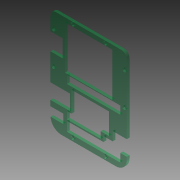
# Autodesk Inventor part: beagle_spacer_top
Saved by Autodesk Inventor 2014 (Build 180170000, 170)
## iProperties
Created: 2013-06-20
Part Number: beagle_spacer_top
Document SubType Name: Modeling
Designer: Administrator
Density: 1 g/cm^3
Mass: 13.5107 g
Surface Area: 121.813 cm^2
Volume: 13.5107 cm^3
Material: Generic
Appearance: Clear - Green 1
Author: Administrator
Autodesk Inventor part; units mm, degrees
ref_plane "YZ Plane" through (0, 0, 0) normal (1, 0, 0) x (0, 1, 0)
ref_plane "XZ Plane" through (0, 0, 0) normal (0, 1, 0) x (-1, 0, 0)
ref_plane "XY Plane" through (0, 0, 0) normal (0, 0, 1) x (1, 0, 0)
sketch "Sketch1" plane through (0, 0, 0) normal (0, 0, 1) x (1, 0, 0)
  line L0 (9.8795, 48.1994) -> (9.8795, -53.4006)
  line L1 (16.2295, 54.5494) -> (92.4295, 54.5494)
  line L2 (98.7795, 48.1994) -> (98.7795, -53.4006)
  line L3 (22.5795, -66.1006) -> (86.0795, -66.1006)
  arc A0 (9.8795, -53.4006) -> (22.5795, -66.1006) centre (22.5795, -53.4006) ccw
  arc A1 (16.2295, 54.5494) -> (9.8795, 48.1994) centre (16.2295, 48.1994) ccw
  arc A2 (98.7795, 48.1994) -> (92.4295, 54.5494) centre (92.4295, 48.1994) ccw
  arc A3 (86.0795, -66.1006) -> (98.7795, -53.4006) centre (86.0795, -53.4006) ccw
  point P0 (0, 0)
  dimension "d0" = 12.7
  dimension "d1" = 6.35
  dimension "d2" = 120.65
  dimension "d3" = 88.9
  constraints: 8 end point, 8 point on circle, 8 tangent, 4 centre point, 2 equal radius, 1 horizontal, 1 vertical
  measures "d0" radius of A0
  measures "d1" radius of A1
  measures "d2" distance between parallel lines of L3 L1
  measures "d3" distance between parallel lines of L2 L0
extrude "Extrusion1" add sketch "Sketch1" along normal blind 3.175
sketch "Sketch2" plane through (0, 0, 3.175) normal (0, 0, 1) x (1, 0, 0)
  line L0 (9.8795, -53.4006) -> (9.8795, 48.1994) projected
  line L1 (98.7795, 48.1994) -> (98.7795, -53.4006) projected
  line L2 (16.2295, 54.5494) -> (92.4295, 54.5494) projected
  line L3 (26.6435, 49.4694) -> (82.0155, 49.4694)
  line L4 (82.0155, 49.4694) -> (82.0155, -1.3306)
  line L5 (82.0155, -1.3306) -> (26.6435, -1.3306)
  line L6 (26.6435, -1.3306) -> (26.6435, 49.4694)
  point P0 (0, 0)
  dimension "d13" = 16.764
  dimension "d14" = 16.764
  dimension "d15" = 5.08
  dimension "d16" = 55.88
  constraints: 8 end point
  measures "d13" distance between parallel lines of L0 L6
  measures "d14" distance between parallel lines of L1 L4
  measures "d15" distance between parallel lines of L2 L3
  measures "d16" distance between parallel lines of L5 L2
extrude "Extrusion2" cut sketch "Sketch2" against normal through all
sketch "Sketch3" plane through (0, 0, 3.175) normal (0, 0, 1) x (1, 0, 0)
  line L0 (9.8795, -53.4006) -> (9.8795, 48.1994) projected
  line L1 (86.0795, -66.1006) -> (22.5795, -66.1006) projected
  line L2 (9.8795, -19.4408) -> (32.7395, -19.4408)
  line L3 (32.7395, -19.4408) -> (32.7395, -37.2208)
  line L4 (32.7395, -37.2208) -> (9.8795, -37.2208)
  point P0 (0, 0)
  dimension "d20" = 28.8798
  dimension "d21" = 46.6598
  dimension "d22" = 22.86
  constraints: 6 end point, 2 point on line
  measures "d20" distance between parallel lines of L4 L1
  measures "d21" distance between parallel lines of L1 L2
  measures "d22" distance between parallel lines of L3 L0
extrude "Extrusion3" cut sketch "Sketch3" against normal through all
sketch "Sketch4" plane through (0, 0, 3.175) normal (0, 0, 1) x (1, 0, 0)
  line L0 (9.8795, -53.4006) -> (9.8795, -37.2208) projected
  arc A0 (9.8795, -53.4006) -> (22.5795, -66.1006) centre (22.5795, -53.4006) ccw projected
  line L1 (86.0795, -66.1006) -> (22.5795, -66.1006) projected
  line L2 (24.8655, -43.5708) -> (24.8655, -54.1626)
  line L3 (24.8655, -43.5708) -> (9.8795, -43.5708)
  line L4 (24.8655, -54.1626) -> (9.9024, -54.1626)
  point P0 (0, 0)
  dimension "d26" = 22.5298
  dimension "d27" = 14.986
  dimension "d28" = 11.938
  constraints: 6 end point, 1 horizontal, 1 point on circle, 1 point on line, 1 vertical
  measures "d26" distance between parallel lines of L1 L3
  measures "d27" distance between parallel lines of L0 L2
  measures "d28" distance between parallel lines of L1 L4
extrude "Extrusion4" cut sketch "Sketch4" against normal through all
sketch "Sketch5" plane through (0, 0, 3.175) normal (0, 0, 1) x (1, 0, 0)
  line L0 (86.0795, -66.1006) -> (22.5795, -66.1006) projected
  line L1 (9.8795, -19.4408) -> (9.8795, 48.1994) projected
  line L2 (9.8795, -43.5708) -> (9.8795, -37.2208) projected
  line L3 (28.9295, -2.1688) -> (91.1595, -2.1688)
  line L4 (91.1595, -2.1688) -> (91.1595, -11.5668)
  line L5 (91.1595, -11.5668) -> (28.9295, -11.5668)
  line L6 (28.9295, -11.5668) -> (28.9295, -2.1688)
  line L7 (28.9295, -50.4288) -> (91.1595, -50.4288)
  line L8 (91.1595, -50.4288) -> (91.1595, -59.8268)
  line L9 (91.1595, -59.8268) -> (28.9295, -59.8268)
  line L10 (28.9295, -59.8268) -> (28.9295, -50.4288)
  point P0 (0, 0)
  dimension "d31" = 54.5338
  dimension "d32" = 9.398
  dimension "d33" = 62.23
  dimension "d34" = 19.05
  dimension "d35" = 19.05
  dimension "d36" = 6.2738
  constraints: 16 end point, 2 equal length
  measures "d31" distance between parallel lines of L0 L5
  measures "d32" distance between parallel lines of L3 L5
  measures "d33" distance of L4.end L5.end
  measures "d34" distance between parallel lines of L1 L6
  measures "d35" distance between parallel lines of L2 L10
  measures "d36" distance between parallel lines of L9 L0
extrude "Extrusion5" cut sketch "Sketch5" against normal through all
sketch "Sketch6" plane through (0, 0, 3.175) normal (0, 0, 1) x (1, 0, 0)
  line L0 (71.6015, -11.5668) -> (28.9295, -11.5668)
  line L1 (28.9295, -50.4288) -> (71.6015, -50.4288)
  line L2 (71.6015, -50.4288) -> (71.6015, -11.5668)
  line L3 (28.9295, -59.8268) -> (28.9295, -50.4288) projected
  line L4 (28.9295, -11.5668) -> (28.9295, -50.4288)
  line L5 (28.9295, -47.2538) -> (68.4265, -47.2538)
  line L6 (9.8795, -19.4408) -> (32.7395, -19.4408) projected
  line L7 (32.7395, -19.4408) -> (32.7395, -37.2208) projected
  line L8 (32.7395, -37.2208) -> (9.8795, -37.2208) projected
  line L9 (28.9295, -17.8533) -> (34.327, -17.8533)
  line L10 (34.327, -17.8533) -> (34.327, -38.8083)
  line L11 (34.327, -38.8083) -> (28.9295, -38.8083)
  line L12 (91.1595, -11.5668) -> (28.9295, -11.5668) projected
  line L13 (28.9295, -50.4288) -> (91.1595, -50.4288) projected
  line L14 (91.1595, -50.4288) -> (91.1595, -42.8088)
  line L15 (91.1595, -42.8088) -> (71.6015, -42.8088)
  line L16 (28.9295, -14.7418) -> (71.6015, -14.7418)
  line L17 (28.9295, -48.8413) -> (71.6015, -48.8413)
  line L18 (68.4265, -47.2538) -> (68.4265, -39.6338)
  line L19 (68.4265, -39.6338) -> (71.6015, -39.6338)
  line L20 (91.1595, -50.4288) -> (71.6015, -50.4288)
  line L21 (98.7795, 48.1994) -> (98.7795, -53.4006) projected
  line L22 (34.327, -17.8533) -> (34.327, -14.7418)
  point P0 (0, 0)
  dimension "d46" = 3.175
  dimension "d49" = 1.5875
  dimension "d50" = 1.5875
  dimension "d51" = 1.5875
  dimension "d54" = 7.62
  dimension "d55" = 3.175
  dimension "d57" = 1.5875
  dimension "d58" = 3.175
  dimension "d61" = 3.175
  dimension "d72" = 27.178
  constraints: 32 end point, 11 point on line, 5 vertical, 2 collinear
  measures "d46" distance between parallel lines of L1 L5
  measures "d49" distance between parallel lines of L8 L11
  measures "d50" distance between parallel lines of L10 L7
  measures "d51" distance between parallel lines of L6 L9
  measures "d54" distance between parallel lines of L13 L15
  measures "d55" distance between parallel lines of L12 L16
  measures "d57" distance between parallel lines of L1 L17
  measures "d58" distance between parallel lines of L15 L19
  measures "d61" distance between parallel lines of L2 L18
  measures "d72" distance between parallel lines of L21 L2
extrude "Extrusion11" cut sketch "Sketch6" against normal through all contours L2 L19 L18 L5 L4 L11 L10 L22 L16 | L15 L14 L13 L2 | L2 L1 L4 L17
sketch "Sketch7" plane through (0, 0, 3.175) normal (0, 0, 1) x (1, 0, 0)
  line L0 (71.6015, -14.7418) -> (71.6015, -39.6338) projected
  line L1 (71.6015, -14.7418) -> (77.9515, -14.7418)
  line L2 (77.9515, -14.7418) -> (77.9515, -39.6338)
  line L3 (77.9515, -39.6338) -> (71.6015, -39.6338)
  point P0 (0, 0)
  dimension "d64" = 6.35
  constraints: 6 end point, 2 horizontal
  measures "d64" distance between parallel lines of L2 L0
extrude "Extrusion12" cut sketch "Sketch7" against normal through all
sketch "Sketch8" plane through (0, 0, 3.175) normal (0, 0, 1) x (1, 0, 0)
  line L0 (86.0795, -66.1006) -> (22.5795, -66.1006) projected
  line L1 (98.7795, 48.1994) -> (98.7795, -53.4006) projected
  line L2 (82.2695, -32.3948) -> (98.7795, -32.3948)
  line L3 (98.7795, -32.3948) -> (98.7795, -50.1748)
  line L4 (98.7795, -50.1748) -> (82.2695, -50.1748)
  line L5 (82.2695, -50.1748) -> (82.2695, -32.3948)
  point P0 (0, 0)
  dimension "d67" = 15.9258
  dimension "d68" = 17.78
  dimension "d69" = 16.51
  constraints: 8 end point, 1 collinear, 1 horizontal, 1 vertical
  measures "d67" distance between parallel lines of L0 L4
  measures "d68" distance of L4.end L2.start
  measures "d69" distance of L2.start L2.end
extrude "Extrusion13" cut sketch "Sketch8" against normal through all
sketch "Sketch9" plane through (0, 0, 3.175) normal (0, 0, 1) x (1, 0, 0)
  line L0 (98.7795, 48.1994) -> (98.7795, -32.3948) projected
  line L1 (16.2295, 54.5494) -> (92.4295, 54.5494) projected
  line L2 (9.8795, -19.4408) -> (9.8795, 48.1994) projected
  line L3 (86.0795, -66.1006) -> (22.5795, -66.1006) projected
  line L4 (36.2694, 49.7107) -> (34.2897, 49.7107)
  line L5 (34.2897, 49.7107) -> (33.2998, 51.4252)
  line L6 (33.2998, 51.4252) -> (34.2897, 53.1397)
  line L7 (34.2897, 53.1397) -> (36.2694, 53.1397)
  line L8 (36.2694, 53.1397) -> (37.2593, 51.4252)
  line L9 (37.2593, 51.4252) -> (36.2694, 49.7107)
  line L10 (75.3593, 51.4252) -> (74.3694, 49.7107)
  line L11 (74.3694, 49.7107) -> (72.3897, 49.7107)
  line L12 (72.3897, 49.7107) -> (71.3998, 51.4252)
  line L13 (71.3998, 51.4252) -> (72.3897, 53.1397)
  line L14 (72.3897, 53.1397) -> (74.3694, 53.1397)
  line L15 (74.3694, 53.1397) -> (75.3593, 51.4252)
  line L16 (97.3698, 34.5095) -> (95.6553, 33.5197)
  line L17 (95.6553, 33.5197) -> (93.9408, 34.5095)
  line L18 (93.9408, 34.5095) -> (93.9408, 36.4893)
  line L19 (93.9408, 36.4893) -> (95.6553, 37.4791)
  line L20 (95.6553, 37.4791) -> (97.3698, 36.4893)
  line L21 (97.3698, 36.4893) -> (97.3698, 34.5095)
  line L22 (37.2593, -62.9764) -> (36.2694, -64.6909)
  line L23 (36.2694, -64.6909) -> (34.2897, -64.6909)
  line L24 (34.2897, -64.6909) -> (33.2998, -62.9764)
  line L25 (33.2998, -62.9764) -> (34.2897, -61.2619)
  line L26 (34.2897, -61.2619) -> (36.2694, -61.2619)
  line L27 (36.2694, -61.2619) -> (37.2593, -62.9764)
  line L28 (75.3593, -62.9764) -> (74.3694, -64.6909)
  line L29 (74.3694, -64.6909) -> (72.3897, -64.6909)
  line L30 (72.3897, -64.6909) -> (71.3998, -62.9764)
  line L31 (71.3998, -62.9764) -> (72.3897, -61.2619)
  line L32 (72.3897, -61.2619) -> (74.3694, -61.2619)
  line L33 (74.3694, -61.2619) -> (75.3593, -62.9764)
  line L34 (97.3698, -3.5905) -> (95.6553, -4.5803)
  line L35 (95.6553, -4.5803) -> (93.9408, -3.5905)
  line L36 (93.9408, -3.5905) -> (93.9408, -1.6107)
  line L37 (93.9408, -1.6107) -> (95.6553, -0.6209)
  line L38 (95.6553, -0.6209) -> (97.3698, -1.6107)
  line L39 (97.3698, -1.6107) -> (97.3698, -3.5905)
  line L40 (14.7182, 34.5095) -> (13.0037, 33.5197)
  line L41 (13.0037, 33.5197) -> (11.2892, 34.5095)
  line L42 (11.2892, 34.5095) -> (11.2892, 36.4893)
  line L43 (11.2892, 36.4893) -> (13.0037, 37.4791)
  line L44 (13.0037, 37.4791) -> (14.7182, 36.4893)
  line L45 (14.7182, 36.4893) -> (14.7182, 34.5095)
  line L46 (14.7182, -1.6107) -> (14.7182, -3.5905)
  line L47 (14.7182, -3.5905) -> (13.0037, -4.5803)
  line L48 (13.0037, -4.5803) -> (11.2892, -3.5905)
  line L49 (11.2892, -3.5905) -> (11.2892, -1.6107)
  line L50 (11.2892, -1.6107) -> (13.0037, -0.6209)
  line L51 (13.0037, -0.6209) -> (14.7182, -1.6107)
  point P0 (0, 0)
  point P1 (35.2795, 51.4252)
  point P2 (73.3795, 51.4252)
  point P3 (95.6553, 35.4994)
  point P4 (35.2795, -62.9764)
  point P5 (73.3795, -62.9764)
  point P6 (95.6553, -2.6006)
  point P7 (13.0037, 35.4994)
  point P8 (13.0037, -2.6006)
  dimension "d73" = 3.429
  dimension "d74" = 3.1242
  dimension "d75" = 3.1242
  dimension "d76" = 3.1242
  dimension "d77" = 3.1242
  dimension "d78" = 25.4
  dimension "d79" = 19.05
  dimension "d80" = 38.1
  dimension "d81" = 38.1
  constraints: 96 end point, 7 equal length, 4 horizontal, 4 horizontal alignment, 4 vertical, 4 vertical alignment, 104 other
  measures "d73" distance between parallel lines of L7 L4
  measures "d74" distance from line of L1 point (35.28, 51.425)
  measures "d75" distance from line of L2 point (13.004, 35.499)
  measures "d76" distance from line of L0 point (95.655, 35.499)
  measures "d77" distance from line of L3 point (35.28, -62.976)
  measures "d78" distance from line of L2 point (35.28, 51.425)
  measures "d79" distance from line of L1 point (13.004, 35.499)
  measures "d80" distance of point (13.004, -2.601) point (13.004, 35.499)
  measures "d81" distance of point (73.38, 51.425) point (35.28, 51.425)
extrude "Extrusion14" cut sketch "Sketch9" against normal through all
sketch "Sketch10" plane through (0, 0, 0) normal (0, 0, -1) x (-1, 0, 0)
  line L0 (-11.2892, 36.4893) -> (-11.2892, 34.5095) projected
  line L1 (-9.8795, 48.1994) -> (-9.8795, -19.4408) projected
  line L2 (-26.6435, 49.4694) -> (-26.6435, -1.3306) projected
  line L3 (-24.1035, 32.11) -> (-24.1035, 11.79)
  line L4 (-24.1035, 32.11) -> (-9.8795, 32.11)
  line L5 (-24.1035, 11.79) -> (-9.8795, 11.79)
  point P0 (-13.0037, 33.5197)
  point P1 (0, 0)
  dimension "d84" = 2.54
  dimension "d86" = 1.4097
  dimension "d87" = 1.4097
  dimension "d88" = 20.32
  constraints: 6 end point, 2 point on line, 1 horizontal, 1 vertical
  measures "d84" distance between parallel lines of L2 L3
  measures "d86" distance between parallel lines of L1 L0
  measures "d87" distance from line of point (-13.004, 33.52) L4
  measures "d88" distance between parallel lines of L4 L5
extrude "Extrusion15" cut sketch "Sketch10" against normal through all
equation "\"d14\" = d13"
equation "\"d35\" = d34"
equation "\"d87\" = d86"
body "Solid1"
